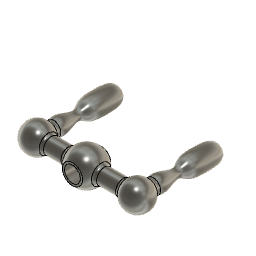
Double Crank (Autodesk Fusion 360 design; units mm, degrees)
Autodesk Fusion 360 part; units mm, degrees
sketch "Sketch1" plane through (0, 0, 0) normal (0, 0, 1) x (1, 0, 0)
  line L0 (-3.96875, 7.14375) -> (-5.020116, 7.14375)
  line L1 (-3.96875, -7.14375) -> (-5.020116, -7.14375)
  arc A0 (-5.020116, 7.14375) -> (-5.020116, -7.14375) centre (0, 0) ccw
  line L2 (-3.96875, 7.14375) -> (-3.96875, -7.14375)
  dimension "d1" = 17.4625
  dimension "d2" = 7.14375
  dimension "d3" = 14.2875
  dimension "d4" = 3.96875
  constraint coincident A0.centre origin
  constraint horizontal L0
  constraint horizontal L1
  constraint perpendicular L0 L2
  measures "d1" diameter of A0
  measures "d2" distance of A0.centre L0
  measures "d3" distance of L0 L1
  measures "d4" distance of A0.centre L2
revolve "Revolve1" add sketch "Sketch1" angle 360 about axis through (0, 1.75, 0) along (0, 1, 0) contours L0 L1 A0 L2 picked at (-5.548347, -0.214335) makes body 1
ref_plane "WorkPlane1" through (25.4, 0, 0) normal (1, 0, 0) x (0, 1, 0)
sketch "Sketch2" plane through (25.4, 0, 0) normal (1, 0, 0) x (0, 1, 0)
  circle A0 centre (0, 0) radius 3.96875
  dimension "d8" = 7.9375
  constraint coincident A0.centre origin
  measures "d8" diameter of A0
extrude "Extrude1" add sketch "Sketch2" against normal blind 50.8 separate body contours A0 picked at (0.431587, 1.004829) makes body 2
ref_plane "WorkPlane3" through (0, -7.14375, 0) normal (0, -1, 0) x (1, 0, 0)
sketch "Sketch3" plane through (0, -7.14375, 0) normal (0, -1, 0) x (1, 0, 0)
  circle A0 centre (0, 0) radius 3.96875
  dimension "d11" = 7.9375
  constraint coincident A0.centre origin
  measures "d11" diameter of A0
extrude "Extrude2" cut sketch "Sketch3" against normal through all contours A0 picked at (0.431587, 1.004829) bodies 2
combine "Combine1" operation add target body 2 tool bodies 1
fillet "Fillet1" radius 2 2 edges at (7.77713, -3.700174, -1.435161) (-7.77713, -3.700174, 1.435161) on bodies 2
ref_plane "WorkPlane5" through (24.60625, 0, 0) normal (1, 0, 0) x (0, 1, 0)
ref_plane "WorkPlane6" through (-24.60625, 0, 0) normal (1, 0, 0) x (0, 1, 0)
sphere "SpherePrimitive1" add diameter 14.2875 placed x (0, 1, 0) y (0, 0, 1) z (1, 0, 0) at (25.4, 0, 0) bodies 2
sphere "SpherePrimitive2" add diameter 14.2875 placed x (0, 1, 0) y (0, 0, 1) z (1, 0, 0) at (-24.60625, 0, 0) bodies 2
fillet "Fillet2" radius 2 2 edges at (19.460119, -3.700174, 1.435161) (-18.666369, -3.700174, -1.435161) on bodies 2
sketch "Sketch6" plane through (0, 0, 0) normal (0, 0, 1) x (1, 0, 0)
  spline S0 degree 5 poles (25.426481, 3.708329) (25.073899, 3.929016) (24.408377, 4.3809) (23.529022, 5.090251) (22.594851, 6.099225) (21.820923, 7.46367) (21.426467, 8.924108) (21.379011, 10.464928) (21.622033, 12.059656) (22.065316, 13.666548) (22.586353, 15.229918) (23.055502, 16.693759) (23.355929, 18.01269) (23.406058, 19.164278) (23.18033, 20.160402) (22.733517, 21.060796) (22.16919, 21.951841) (21.604346, 22.922933) (21.137049, 24.044706) (20.809057, 25.34401) (20.61829, 26.811016) (20.536281, 28.409579) (20.52419, 30.0864) (20.547942, 31.780047) (20.597006, 33.431069) (20.689572, 34.987401) (20.860617, 36.403769) (21.15432, 37.642711) (21.615062, 38.674955) (22.278358, 39.480354) (23.163749, 40.048139) (24.05691, 40.30876) (24.831681, 40.395072) (25.394738, 40.404188) (25.687901, 40.396639) knots 0 0 0 0 0 0 0.03333333 0.06666667 0.1 0.13333333 0.16666667 0.2 0.23333333 0.26666667 0.3 0.33333333 0.36666667 0.4 0.43333333 0.46666667 0.5 0.53333333 0.56666667 0.6 0.63333333 0.66666667 0.7 0.73333333 0.76666667 0.8 0.83333333 0.86666667 0.9 0.93333333 0.96666667 1 1 1 1 1 1
  line L0 (25.687901, 40.396639) -> (25.426481, 3.708329)
  line L1 (25.687901, 40.396639) -> (25.426481, 3.708329)
  spline S1 degree 5 poles (25.426481, 3.708329) (25.073899, 3.929016) (24.408377, 4.3809) (23.529022, 5.090251) (22.594851, 6.099225) (21.820923, 7.46367) (21.426467, 8.924108) (21.379011, 10.464928) (21.622033, 12.059656) (22.065316, 13.666548) (22.586353, 15.229918) (23.055502, 16.693759) (23.355929, 18.01269) (23.406058, 19.164278) (23.18033, 20.160402) (22.733517, 21.060796) (22.16919, 21.951841) (21.604346, 22.922933) (21.137049, 24.044706) (20.809057, 25.34401) (20.61829, 26.811016) (20.536281, 28.409579) (20.52419, 30.0864) (20.547942, 31.780047) (20.597006, 33.431069) (20.689572, 34.987401) (20.860617, 36.403769) (21.15432, 37.642711) (21.615062, 38.674955) (22.278358, 39.480354) (23.163749, 40.048139) (24.05691, 40.30876) (24.831681, 40.395072) (25.394738, 40.404188) (25.687901, 40.396639) knots 0 0 0 0 0 0 0.03333333 0.06666667 0.1 0.13333333 0.16666667 0.2 0.23333333 0.26666667 0.3 0.33333333 0.36666667 0.4 0.43333333 0.46666667 0.5 0.53333333 0.56666667 0.6 0.63333333 0.66666667 0.7 0.73333333 0.76666667 0.8 0.83333333 0.86666667 0.9 0.93333333 0.96666667 1 1 1 1 1 1
  point P0 (21.573, 38.46)
  point P1 (20.541078, 31.019857)
  point P2 (17.727, 0)
  point P3 (21.573, 11.538)
  point P4 (23.331753, 19.193733)
  point P5 (21.573, 23.076)
  point P6 (21.573, 23.076)
  point P7 (21.573, 38.46)
  point P8 (20.541078, 31.019857)
  point P9 (21.573, 11.538)
  point P10 (23.331753, 19.193733)
scale "Scale1" [no effect]
revolve "Revolve2" add sketch "Sketch6" angle 360 about axis through (25.740185, 47.734301, 0) along (-0.00712525, -0.99997462, 0) separate body contours S0 L0 L1 S1 picked at (23.021815, 29.911044) makes body 3
sketch "Sketch7" plane through (0, 0, 0) normal (0, 0, 1) x (1, 0, 0)
  line L0 (-24.312099, 40.396639) -> (-24.573519, 3.708329)
  spline S0 degree 5 poles (-24.573519, 3.708329) (-24.926101, 3.929016) (-25.591623, 4.3809) (-26.470978, 5.090251) (-27.405149, 6.099225) (-28.179077, 7.46367) (-28.573533, 8.924108) (-28.620989, 10.464928) (-28.377967, 12.059656) (-27.934684, 13.666548) (-27.413647, 15.229918) (-26.944498, 16.693759) (-26.644071, 18.01269) (-26.593942, 19.164278) (-26.81967, 20.160402) (-27.266483, 21.060796) (-27.83081, 21.951841) (-28.395654, 22.922933) (-28.862951, 24.044706) (-29.190943, 25.34401) (-29.38171, 26.811016) (-29.463719, 28.409579) (-29.47581, 30.0864) (-29.452058, 31.780047) (-29.402994, 33.431069) (-29.310428, 34.987401) (-29.139383, 36.403769) (-28.84568, 37.642711) (-28.384938, 38.674955) (-27.721642, 39.480354) (-26.836251, 40.048139) (-25.94309, 40.30876) (-25.168319, 40.395072) (-24.605262, 40.404188) (-24.312099, 40.396639) knots 0 0 0 0 0 0 0.03333333 0.06666667 0.1 0.13333333 0.16666667 0.2 0.23333333 0.26666667 0.3 0.33333333 0.36666667 0.4 0.43333333 0.46666667 0.5 0.53333333 0.56666667 0.6 0.63333333 0.66666667 0.7 0.73333333 0.76666667 0.8 0.83333333 0.86666667 0.9 0.93333333 0.96666667 1 1 1 1 1 1
  point P0 (-28.427, 23.076)
  point P1 (-28.427, 38.46)
  point P2 (-29.458922, 31.019857)
  point P3 (-28.427, 11.538)
  point P4 (-26.668247, 19.193733)
revolve "Revolve3" add sketch "Sketch7" angle 360 about axis through (-24.259815, 47.734301, 0) along (-0.00712525, -0.99997462, 0) separate body contours L0 S0 picked at (-26.978185, 29.911044) makes body 4
combine "Combine2" operation add target body 2 tool bodies 4
combine "Combine3" operation add target body 2 tool bodies 3
fillet "Fillet3" radius 2 2 edges at (28.45769, 6.456291, -0.001217) (-21.543805, 6.454037, -0.001213) on bodies 2
